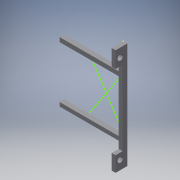
# Autodesk Inventor part: estructura union gusano
Saved by Autodesk Inventor 2016 (Build 200138000, 138)
## iProperties
Created: 2016-08-18
Part Number: estructura union gusano
Material: Generic
Document SubType Name: Modeling
Designer: Admin
Density: 1 g/cm^3
Appearance: Default
Author: Admin
Autodesk Inventor part; units mm, degrees
ref_plane "YZ Plane" through (0, 0, 0) normal (1, 0, 0) x (0, 1, 0)
ref_plane "XZ Plane" through (0, 0, 0) normal (0, 1, 0) x (-1, 0, 0)
ref_plane "XY Plane" through (0, 0, 0) normal (0, 0, 1) x (1, 0, 0)
sketch "Sketch2" plane through (0, 0, 0) normal (1, 0, 0) x (0, 1, 0)
  line L0 (0, 0) -> (-40, 0)
  line L1 (-40, 0) -> (-40, -270)
  line L2 (-40, -270) -> (0, -270)
  line L3 (0, -270) -> (0, 0)
  dimension "d0" = 40
  dimension "d1" = 270
  constraints: 8 end point, 2 parallel, 1 horizontal, 1 perpendicular
  measures "d0" distance of L2.end L1.end
  measures "d1" distance of L1.end L0.end
extrude "Extrusion1" add sketch "Sketch2" along normal blind 10
sketch "Sketch3" plane through (10, 0, 0) normal (1, 0, 0) x (0, 0, -1)
  circle A0 centre (22, -18) radius 7
  line L0 (270, 0) -> (0, 0) projected
  dimension "d4" = 14
  dimension "d10" = 18
  constraints: 1 centre point
  measures "d4" diameter of A0
  measures "d10" distance from line of L0 A0.centre
extrude "Extrusion2" cut sketch "Sketch3" against normal through all
sketch "Sketch4" plane through (10, 0, 0) normal (1, 0, 0) x (0, 0, -1)
  circle A0 centre (247, -18) radius 7
  line L0 (270, 0) -> (0, 0) projected
  dimension "d7" = 14
  dimension "d11" = 18
  constraints: 1 centre point
  measures "d7" diameter of A0
  measures "d11" distance from line of L0 A0.centre
extrude "Extrusion3" cut sketch "Sketch4" against normal through all
sketch "Sketch5" plane through (10, 0, 0) normal (1, 0, 0) x (0, 0, -1)
  line L0 (41.1855, -36.3701) -> (231.1855, -36.3701)
  line L1 (231.1855, -36.3701) -> (231.1855, -14.3701)
  line L2 (231.1855, -14.3701) -> (41.1855, -14.3701)
  line L3 (41.1855, -14.3701) -> (41.1855, -36.3701)
  point P0 (0, 0)
  dimension "d14" = 22
  dimension "d15" = 190
  constraints: 8 end point, 2 parallel, 1 horizontal, 1 perpendicular
  measures "d14" distance between parallel lines of L0 L2
  measures "d15" distance between parallel lines of L1 L3
extrude "Extrusion4" cut sketch "Sketch5" against normal through all
sketch "Sketch15" plane through (10, 0, 0) normal (1, 0, 0) x (0, 0, -1)
  line L0 (135, 10) -> (85, 10)
  line L1 (85, 10) -> (185, 10)
  line L2 (185, 10) -> (231.1855, 0)
  line L3 (270, 0) -> (0, 0) projected
  line L4 (85, 10) -> (41.1855, 0)
  line L5 (41.1855, -36.3701) -> (41.1855, -14.3701) projected
  line L6 (41.1855, -14.3701) -> (85, 0)
  line L7 (185, 0) -> (231.1855, -12.1069)
  point P0 (41.1855, -30)
  dimension "d37" = 50
  dimension "d38" = 100
  constraints: 12 end point, 4 point on line, 1 collinear
  measures "d37" distance of L0.start L0.end
  measures "d38" distance of L0.end L1.end
extrude "Extrusion10" add sketch "Sketch15" against normal blind 10
sketch "Sketch16" plane through (10, 0, 0) normal (1, 0, 0) x (0, 0, -1)
  line L0 (41.1855, -14.3701) -> (231.1855, -14.3701) projected
  line L1 (41.1855, -14.3701) -> (85, -2.2632)
  line L2 (85, -2.2632) -> (185, -2.2632)
  line L3 (85, 10) -> (185, 10) projected
  line L4 (185, -2.2632) -> (231.1855, -14.3701)
  point P0 (0, 0)
  constraints: 6 end point, 1 parallel
extrude "Extrusion11" cut sketch "Sketch16" against normal through all
body "Solid1"
